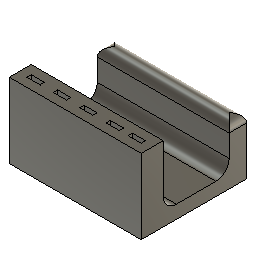
laptop Stand (Autodesk Fusion 360 design; units mm, degrees)
Autodesk Fusion 360 part; units mm, degrees
sketch "Sketch1" plane through (0, 0, 0) normal (0, 0, 1) x (1, 0, 0)
  line L0 (-75, 75) -> (75, 75)
  line L1 (75, 75) -> (75, -25)
  line L2 (75, -25) -> (-75, -25)
  line L3 (-75, -25) -> (-75, 75)
  dimension "d1" = 150
  dimension "d2" = 100
  constraint perpendicular L0 L1
  constraint parallel L0 L2
  constraint parallel L1 L3
  constraint horizontal L0
  measures "d1" distance of L0.start L0.end
  measures "d2" distance of L0.start L2.end
extrude "Extrude1" add sketch "Sketch1" along normal blind 10
sketch "Sketch2" plane through (0, 0, 10) normal (0, 0, 1) x (-1, 0, 0)
  line L0 (75, 25) -> (-75, 25)
  line L1 (-75, 25) -> (-75, -75)
  line L2 (-75, -75) -> (75, -75)
  line L3 (75, -75) -> (75, 25)
  line L4 (-75, 25) -> (75, 25)
  line L5 (75, 25) -> (75, 0)
  line L6 (75, 0) -> (-75, 0)
  line L7 (-75, 0) -> (-75, 25)
  constraint horizontal L4
  constraint vertical L5
  constraint horizontal L6
  constraint vertical L7
  constraint coincident L3 L5.end
  constraint coincident L0.end L1.start
extrude "Extrude2" add sketch "Sketch2" along normal blind 75 contours L0 L1 L3 L4 L5 L6 L7
sketch "Sketch3" plane through (0, 0, 10) normal (0, 0, 1) x (-1, 0, 0)
  line L0 (75, 0) -> (-75, 0)
  line L1 (-75, 0) -> (-75, -75)
  line L2 (-75, -75) -> (75, -75)
  line L3 (75, -75) -> (75, 0)
extrude "Extrude3" add sketch "Sketch3" along normal blind 5
extrude "Extrude4" add 1 faces at (25, 75, 5) along direction (0, 1, 0) blind 20
sketch "Sketch4" plane through (0, 0, 15) normal (0, 0, 1) x (-1, 0, 0)
  line L0 (75, -95) -> (75, 0)
  line L1 (75, 0) -> (-75, 0)
  line L2 (-75, 0) -> (-75, -95)
  line L3 (-75, -95) -> (75, -95)
  line L4 (-75, -75) -> (75, -75)
  line L5 (75, -75) -> (75, -95)
  line L6 (75, -95) -> (-75, -95)
  line L7 (-75, -95) -> (-75, -75)
  constraint horizontal L4
  constraint vertical L5
  constraint horizontal L6
  constraint vertical L7
  constraint coincident L0.start L3.end
  constraint coincident L2 L4.start
extrude "Extrude5" add sketch "Sketch4" along normal blind 50 contours L0 L2 L3 L4 L5 L6 L7
fillet "Fillet1" radius 15 1 edges at (0, 0, 15)
fillet "Fillet2" radius 15 1 edges at (0, 75, 15)
sketch "Sketch5" plane through (0, 0, 85) normal (0, 0, 1) x (-1, 0, 0)
  line L0 (-75, 0) -> (75, 0)
  line L1 (75, 0) -> (75, 25)
  line L2 (75, 25) -> (-75, 25)
  line L3 (-75, 25) -> (-75, 0)
  line L4 (65, 10) -> (50, 10)
  line L5 (50, 10) -> (50, 15)
  line L6 (50, 15) -> (65, 15)
  line L7 (65, 15) -> (65, 10)
  line L8 (35, 10) -> (20, 10)
  line L9 (20, 10) -> (20, 15)
  line L10 (20, 15) -> (35, 15)
  line L11 (35, 15) -> (35, 10)
  line L12 (5, 10) -> (-10, 10)
  line L13 (-10, 10) -> (-10, 15)
  line L14 (-10, 15) -> (5, 15)
  line L15 (5, 15) -> (5, 10)
  line L16 (-25, 10) -> (-40, 10)
  line L17 (-40, 10) -> (-40, 15)
  line L18 (-40, 15) -> (-25, 15)
  line L19 (-25, 15) -> (-25, 10)
  line L20 (-50, 10) -> (-65, 10)
  line L21 (-65, 10) -> (-65, 15)
  line L22 (-65, 15) -> (-50, 15)
  line L23 (-50, 15) -> (-50, 10)
  constraint horizontal L4
  constraint vertical L5
  constraint horizontal L6
  constraint vertical L7
  constraint horizontal L8
  constraint vertical L9
  constraint horizontal L10
  constraint vertical L11
  constraint horizontal L12
  constraint vertical L13
  constraint horizontal L14
  constraint vertical L15
  constraint horizontal L16
  constraint vertical L17
  constraint horizontal L18
  constraint vertical L19
  constraint horizontal L20
  constraint vertical L21
  constraint horizontal L22
  constraint vertical L23
extrude "Extrude6" add sketch "Sketch5" along normal blind 5 contours L4 L5 L6 L7 | L8 L9 L10 L11 | L12 L13 L14 L15 | L16 L17 L18 L19 | L20 L21 L22 L23
fillet "Fillet3" radius 10 1 faces at (-25, 88.3333, 65)
extrude "Extrude7" cut 1 faces at (0, -11.6667, 90) along direction (0, 0, -1) blind 10
extrude "Extrude8" cut 1 faces at (-30, -11.6667, 90) along direction (0, 0, -1) blind 10
extrude "Extrude9" cut 1 faces at (-60, -11.6667, 90) along direction (0, 0, -1) blind 10
extrude "Extrude10" cut 1 faces at (30, -11.6667, 90) along direction (0, 0, -1) blind 10
extrude "Extrude11" cut 1 faces at (55, -11.6667, 90) along direction (0, 0, -1) blind 10
